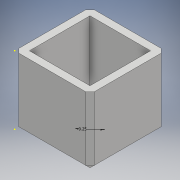
# Autodesk Inventor part: cuvette holder lid
Saved by Autodesk Inventor 2017 (Build 210142000, 142)
## iProperties
Created: 2018-08-10
Part Number: cuvette holder lid
Material: Generic
Document SubType Name: Modeling
Designer: qwertyuiop1
Density: 1 g/cm^3
Appearance: Default
Author: qwertyuiop1
Autodesk Inventor part; units mm, degrees
ref_plane "YZ Plane" through (0, 0, 0) normal (1, 0, 0) x (0, 1, 0)
ref_plane "XZ Plane" through (0, 0, 0) normal (0, 1, 0) x (-1, 0, 0)
ref_plane "XY Plane" through (0, 0, 0) normal (0, 0, 1) x (1, 0, 0)
sketch "Sketch1" plane through (0, 0, 0) normal (0, 0, 1) x (1, 0, 0)
  line L0 (0, 0) -> (33.25, 0)
  line L1 (33.25, 0) -> (33.25, 33.25)
  line L2 (33.25, 33.25) -> (0, 33.25)
  line L3 (0, 33.25) -> (0, 0)
  dimension "d0" = 33.25
  dimension "d1" = 33.25
  constraints: 8 end point, 2 parallel, 1 horizontal, 1 perpendicular
  measures "d0" distance of L2.end L1.end
  measures "d1" distance of L1.end L0.end
extrude "Extrusion1" add sketch "Sketch1" along normal blind 30
sketch "Sketch2" plane through (0, 0, 30) normal (0, 0, 1) x (1, 0, 0)
  point P0 (0, 0)
sketch "Sketch3" plane through (0, 0, 30) normal (0, 0, 1) x (1, 0, 0)
  line L0 (3.25, 3.25) -> (30, 3.25)
  line L1 (30, 3.25) -> (30, 30)
  line L2 (30, 30) -> (3.25, 30)
  line L3 (3.25, 30) -> (3.25, 3.25)
  line L4 (33.25, 0) -> (33.25, 33.25) projected
  line L5 (0, 0) -> (33.25, 0)
  line L6 (33.25, 0) -> (33.25, 33.25)
  line L7 (33.25, 33.25) -> (0, 33.25)
  line L8 (0, 33.25) -> (0, 0)
  dimension "d4" = 26.75
  dimension "d5" = 26.75
  constraints: 16 end point, 4 parallel, 2 horizontal, 2 perpendicular
  measures "d4" distance of L2.end L1.end
  measures "d5" distance of L1.end L0.end
extrude "Extrusion2" cut sketch "Sketch3" against normal blind 26.75 contours L3 L2 L1 L0
chamfer "Chamfer1" distance 1.875 angle 45 8 edges at (33.25, 33.25, 15) (33.25, 0, 15) (0, 33.25, 15) (0, 0, 15) (0, 16.625, 0) (16.625, 33.25, 0) (16.625, 0, 0) (33.25, 16.625, 0)
sketch "Sketch4" plane through (0, 0, 0) normal (0, 0, -1) x (-1, 0, 0)
  circle A0 centre (-16.625, 16.625) radius 4.625
  point P0 (0, 0)
  dimension "d11" = 9.25
  constraints: 1 centre point
  measures "d11" diameter of A0
body "Solid1"
